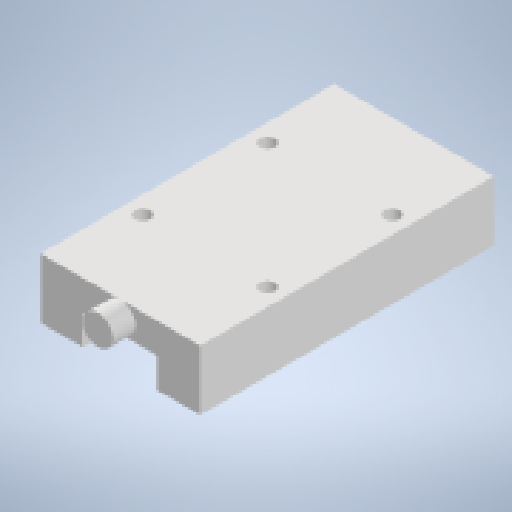
# Autodesk Inventor part: MGN15H-Carrier
Saved by Autodesk Inventor 2023 (Build 270158000, 158)
## iProperties
Created: 2022-04-29
Part Number: MGN15H-Carrier
Material: Generic
Document SubType Name: Modeling
Designer: plebbb
Density: 1 g/cm^3
Appearance: Default
Author: plebbb
Autodesk Inventor part; units mm, degrees
ref_plane "YZ Plane" through (0, 0, 0) normal (1, 0, 0) x (0, 1, 0)
ref_plane "XZ Plane" through (0, 0, 0) normal (0, 1, 0) x (-1, 0, 0)
ref_plane "XY Plane" through (0, 0, 0) normal (0, 0, 1) x (1, 0, 0)
sketch "Sketch1" plane through (0, 0, 0) normal (0, 0, 1) x (1, 0, 0)
  line L0 (0, 12) -> (0, 0)
  line L1 (0, 0) -> (8.5, 0)
  line L2 (8.5, 0) -> (8.5, 6)
  line L3 (8.5, 6) -> (23.5, 6)
  line L4 (23.5, 6) -> (23.5, 0)
  line L5 (23.5, 0) -> (32, 0)
  line L6 (32, 0) -> (32, 12)
  line L7 (32, 12) -> (0, 12)
  dimension "d0" = 32
  dimension "d1" = 12
  dimension "d2" = 8.5
  dimension "d3" = 6
  constraints: 16 end point, 6 perpendicular, 2 point on line, 1 coincident, 1 collinear, 1 vertical
  measures "d0" distance of L6.end L0.start
  measures "d1" distance of L0.start L0.end
  measures "d2" distance of L0.end L1.end
  measures "d3" distance of L1.end L2.end
extrude "Extrusion1" add sketch "Sketch1" along normal blind 58.8
sketch "Sketch2" plane through (0, 12, 0) normal (0, 1, 0) x (1, 0, 0)
  line L0 (3.5, -41.9) -> (28.5, -41.9) construction
  line L1 (28.5, -41.9) -> (28.5, -16.9) construction
  line L2 (28.5, -16.9) -> (3.5, -16.9) construction
  line L3 (3.5, -16.9) -> (3.5, -41.9) construction
  circle A0 centre (3.5, -41.9) radius 1.5
  circle A1 centre (3.5, -16.9) radius 1.5
  circle A2 centre (28.5, -41.9) radius 1.5
  circle A3 centre (28.5, -16.9) radius 1.5
  line L4 (32, -58.8) -> (0, -58.8) construction
  line L5 (32, 0) -> (0, 0) construction
  line L6 (16, -41.9) -> (16, -58.8) construction
  line L7 (16, -16.9) -> (16, 0) construction
  dimension "d6" = 3
  dimension "d7" = 25
  dimension "d8" = 25
  constraints: 12 end point, 4 centre point, 4 coincident, 4 midpoint, 3 equal radius, 2 parallel, 2 vertical, 1 collinear, 1 horizontal, 1 perpendicular
  measures "d6" diameter of A0
  measures "d7" distance of L2.end L0.start
  measures "d8" distance of L1.end L2.end
extrude "Extrusion2" cut sketch "Sketch2" against normal blind 4
sketch "Sketch3" plane through (0, 0, 58.8) normal (0, 0, 1) x (1, 0, 0)
  line L0 (8.5, 6) -> (23.5, 6) projected
  line L1 (32, 12) -> (0, 12) projected
  circle A0 centre (16, 9) radius 3
  point P0 (0, 0)
  point P1 (16, 12)
  dimension "d11" = 6
  constraints: 1 centre point, 1 midpoint, 1 tangent, 1 vertical alignment
  measures "d11" diameter of A0
extrude "Extrusion3" add sketch "Sketch3" along normal blind 4.5
body "Solid1"
